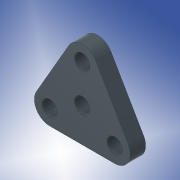
# Autodesk Inventor part: Carrier
Saved by Autodesk Inventor 2017 SP1 (Build 210196100, 196)
## iProperties
Created: 2017-07-05
Part Number: Carrier
Material: ABS Plastic
Document SubType Name: Modeling
Designer: Zach
Density: 1.06 g/cm^3
Appearance: CR Dark Blue
Author: Zach
Autodesk Inventor part; units mm, degrees
ref_plane "YZ Plane" through (0, 0, 0) normal (1, 0, 0) x (0, 1, 0)
ref_plane "XZ Plane" through (0, 0, 0) normal (0, 1, 0) x (-1, 0, 0)
ref_plane "XY Plane" through (0, 0, 0) normal (0, 0, 1) x (1, 0, 0)
sketch "Sketch1" plane through (0, 0, 0) normal (0, 0, 1) x (1, 0, 0)
  line L0 (0, 0) -> (21, 36.3731) construction
  line L1 (0, 0) -> (42, 0) construction
  line L2 (42, 0) -> (21, 36.3731) construction
  circle A0 centre (21, 36.3731) radius 5
  circle A1 centre (42, 0) radius 5
  circle A2 centre (0, 0) radius 5
  circle A3 centre (21, 36.3731) radius 10 construction
  circle A4 centre (42, 0) radius 10 construction
  circle A5 centre (0, 0) radius 10 construction
  line L3 (-8.6603, 5) -> (12.3397, 41.3731)
  line L4 (29.6603, 41.3731) -> (50.6603, 5)
  line L5 (42, -10) -> (0, -10)
  arc A6 (-8.6603, 5) -> (0, -10) centre (0, 0) ccw
  arc A7 (29.6603, 41.3731) -> (12.3397, 41.3731) centre (21, 36.3731) ccw
  arc A8 (42, -10) -> (50.6603, 5) centre (42, 0) ccw
  circle A9 centre (21, 12.1244) radius 5
  line L6 (21, 12.1244) -> (21, -10) construction
  line L7 (21, 12.1244) -> (40.1603, 23.1865) construction
  line L8 (21, 12.1244) -> (1.8397, 23.1865) construction
  point P0 (31.5, 18.1865)
  dimension "d0" = 42
  dimension "d2" = 42
  dimension "d3" = 10
  dimension "d4" = 10
  dimension "d5" = 10
  dimension "d6" = 5
  dimension "d7" = 5
  dimension "d8" = 5
  dimension "d11" = 10
  constraints: 18 end point, 12 point on circle, 10 centre point, 10 tangent, 4 midpoint, 3 coincident, 1 concentric, 1 equal length, 1 horizontal, 1 point on line, 1 vertical
  measures "d0" distance of L0.start L0.end
  measures "d2" distance of L1.end L0.end
  measures "d3" diameter of A0
  measures "d4" diameter of A1
  measures "d5" diameter of A2
  measures "d6" radial gap between concentric circles of A0 A3
  measures "d7" radial gap between concentric circles of A1 A4
  measures "d8" radial gap between concentric circles of A2 A5
  measures "d11" diameter of A9
extrude "Extrusion1" add sketch "Sketch1" along normal blind 10
equation "\"d2\" = d0"
body "Solid1"
